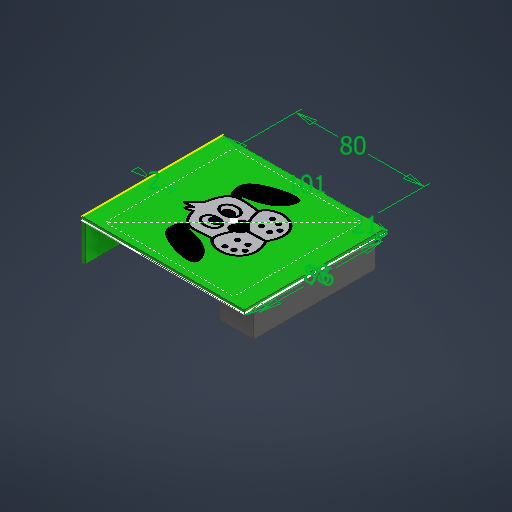
# Autodesk Inventor part: Bitdoglab
Saved by Autodesk Inventor 2027 (Build 310192000, 192)
## iProperties
Created: 2026-10-02
Part Number: Bitdoglab
Material: Genérico
Document SubType Name: Modeling
Designer: EspacoMaker
Density: 1 g/cm^3
Appearance: Padrão
Author: EspacoMaker
Autodesk Inventor part; units mm, degrees
ref_plane "YZ Plane" through (0, 0, 0) normal (1, 0, 0) x (0, 1, 0)
ref_plane "XZ Plane" through (0, 0, 0) normal (0, 1, 0) x (-1, 0, 0)
ref_plane "XY Plane" through (0, 0, 0) normal (0, 0, 1) x (1, 0, 0)
sketch "Esboço1" plane through (0, 0, 0) normal (0, 1, 0) x (-1, 0, 0)
  line L0 (50.5, 44) -> (-50.5, 44)
  line L1 (-50.5, 44) -> (-50.5, -44)
  line L2 (-50.5, -44) -> (50.5, -44)
  line L3 (50.5, -44) -> (50.5, 44)
  line L4 (50.5, 44) -> (-50.5, -44) construction
  line L5 (-50.5, 44) -> (50.5, -44) construction
  line L6 (-29.5, 38) -> (-50.5, 38)
  line L7 (-50.5, 38) -> (-50.5, -38)
  line L8 (-50.5, -38) -> (-29.5, -38)
  line L9 (-29.5, -38) -> (-29.5, 38)
  line L10 (-29.5, 38) -> (-50.5, -38) construction
  line L11 (-50.5, 38) -> (-29.5, -38) construction
  line L12 (48.5, -44) -> (48.5, 44)
  point P0 (0, 0)
  point P1 (-40, 0)
  dimension "d0" = 101
  dimension "d1" = 88
  dimension "d2" = 21
  dimension "d3" = 76
  dimension "d4" = 2
  constraints: 26 end point, 5 parallel, 4 midpoint, 2 horizontal, 2 perpendicular, 1 collinear, 1 horizontal alignment
  measures "d0" distance of L2.end L1.end
  measures "d1" distance of L1.end L0.end
  measures "d2" distance of L8.end L7.end
  measures "d3" distance of L7.end L6.end
  measures "d4" distance between parallel lines of L3 L12
extrude "Extrusão1" add sketch "Esboço1" along normal blind 2
extrude "Extrusão2" add sketch "Esboço1" against normal blind 23 contours L3 L2 L12 L0
extrude "Extrusão3" add sketch "Esboço1" against normal blind 17 contours L6 L9 L8 L1
ref_plane "Plano de trabalho1" through (0, 0, 0) normal (0, 1, 0) x (1, 0, 0)
split_face "Dividir1"
sketch "Esboço2" plane through (0, 2, 0) normal (0, 1, 0) x (1, 0, 0)
  line L0 (-50.5, 44) -> (-50.5, -44) projected
  line L1 (-40, -40) -> (-40, 40) construction
  line L2 (-40, 40) -> (40, 40) construction
  line L3 (40, 40) -> (40, -40) construction
  line L4 (40, -40) -> (-40, -40) construction
  line L5 (-40, -40) -> (40, 40) construction
  point P0 (0, 0)
  point P1 (0, 0)
  dimension "d25" = 80
  constraints: 4 end point, 1 coincident, 1 midpoint, 1 vertical, 2 other
  measures "d25" distance of L1.end L2.end
